junk 2_v2 (Autodesk Fusion 360 design; units mm, degrees)
Autodesk Fusion 360 part; units mm, degrees
note: some values were not read from the file. Chosen so that the rebuilt part matches the saved one: which bodies a step acts on.
sketch "pump stamp sketch" plane through (0, 0, 0) normal (0, 0, 1) x (1, 0, 0)
  circle A0 centre (0, 0) radius 15
  circle A1 centre (-24.5, 0) radius 1.5
  circle A2 centre (-15.5, 15.5) radius 1.5
  circle A3 centre (15.5, 15.5) radius 1.5
  circle A4 centre (-15.5, -15.5) radius 1.5
  circle A5 centre (15.5, -15.5) radius 1.5
  line L0 (-26, 17) -> (26, 17)
  line L1 (26, 17) -> (26, -17)
  line L2 (26, -17) -> (-26, -17)
  line L3 (-26, -17) -> (-26, 17)
  line L4 (-26, 17) -> (26, -17) construction
  line L5 (26, 17) -> (-26, -17) construction
  circle A6 centre (24.5, 0) radius 1.5
  dimension "d569" = 30
  dimension "d570" = 3
  dimension "d576" = 3
  dimension "d579" = 31
  dimension "d580" = -31
  dimension "d581" = 15.5
  dimension "d582" = 15.5
  dimension "d583" = 52
  dimension "d584" = 34
  dimension "d587" = 49
  dimension "d588" = 0
  constraint horizontal A0.centre A1.centre
  constraint coincident A0.centre origin
  constraint horizontal L0
  constraint perpendicular L0 L1
  constraint parallel L0 L2
  constraint parallel L1 L3
  constraint coincident L4 A0.centre
  constraint coincident L5 A0.centre
  constraint tangent L1 A6
  measures "d569" diameter of A0
  measures "d570" diameter of A1
  measures "d576" diameter of A2
  measures "d581" horizontal distance of A0.centre A2.centre
  measures "d582" vertical distance of A0.centre A2.centre
  measures "d583" distance of L0.start L0.end
  measures "d584" distance of L0.start L2.end
extrude "Extrude Pump Stamp" add sketch "pump stamp sketch" along normal blind 4.175 contours A0 | A1 | A4 | A5 | A6 | A3 | A2 makes body 1 at (-14.0075, -15.3506, 2.7833) makes body 2 at (3.6653, 3.4009, 0) makes body 3 at (16.9925, -15.3506, 2.7833) makes body 4 at (-23.0075, -0.1494, 1.3917) makes body 5 at (16.9925, 15.6494, 2.7833) makes body 6 at (25.9925, -0.1494, 2.7833) makes body 7 at (-14.0075, 15.6494, 2.7833)
sketch " minus 1 mm base" plane through (0, 0, 0) normal (0, 0, 1) x (1, 0, 0)
  line L0 (-41.472, 21.911) -> (35.1129, 21.911)
  line L1 (35.1129, 21.911) -> (35.1129, -26.7494)
  line L2 (35.1129, -26.7494) -> (-41.472, -26.7494)
  line L3 (-41.472, -26.7494) -> (-41.472, 21.911)
  dimension "d591" = 76.5849
  constraint horizontal L0
  constraint vertical L1
  constraint horizontal L2
  constraint vertical L3
  measures "d591" distance of L0.start L0.end
extrude "Extrude The minus 1mm base" add sketch " minus 1 mm base" against normal blind 1 bodies 1 7 2 5 4 6 3
copy_body "CopyPasteBodies13" bodies 1 makes body 8
move_body "Move38" bodies 8 to x (1, 0, 0) y (0, 1, 0) z (0, 0, 1) at (100, 0, 0)
sketch "Sketch18" plane through (0, 0, 0) normal (0, 0, 1) x (1, 0, 0)
  line L0 (42.8223, 34.8293) -> (158.9585, 34.8293)
  line L1 (158.9585, 34.8293) -> (158.9585, -31.3539)
  line L2 (158.9585, -31.3539) -> (42.8223, -31.3539)
  line L3 (42.8223, -31.3539) -> (42.8223, 34.8293)
  dimension "d596" = 116.1362
  constraint horizontal L0
  constraint vertical L1
  constraint horizontal L2
  constraint vertical L3
  measures "d596" distance of L0.start L0.end
extrude "Extrude23" cut sketch "Sketch18" against normal blind 1 bodies 8 makes body 9 at (114.3509, -16.4642, 2.7833) makes body 10 at (125.9925, -0.1494, 2.7833) makes body 11 at (76.9925, -0.1494, 1.3917) makes body 12 at (114.6244, 14.2821, 2.7833) makes body 13 at (103.8315, 5.6199, 4.175) makes body 14 at (85.9925, 15.6494, 2.7833)
equation "fingerWidth = 10 mm"
equation "length = 240 mm"
equation "thickness = 3.175 mm"
equation "height = 60 mm"
equation "toolDiameter = 1.401 mm"
equation "boneCornerToCenter = toolDiameter / 2 / sqrt(2) - 0 * kerf" comment "Best: 2.001 -2*kerf, 0.1;;;Best: 2.001 no kerf and 0.1   OLD+6 kerf at 2.001 Diam and .1 mm"
equation "tempLengthPiecesBottom = ceil(( ( floor(( length - 2 * thickness ) / fingerWidth) - 2 ) - ( ( floor(( length - 2 * thickness ) / fingerWidth) - 2 ) % 2 - 1 ) ))"
equation "lengthCutsBottom = ceil(tempLengthPiecesBottom / 2)"
equation "lengthShoulder = ( length - fingerWidth * tempLengthPiecesBottom ) / 2 - kerf"
equation "depth = 185 mm"
equation "tempDepthPiecesBottom = ceil(( ( floor(( depth - 2 * thickness ) / fingerWidth) - 2 ) - ( ( floor(( depth - 2 * thickness ) / fingerWidth) - 2 ) % 2 - 1 ) ))"
equation "depthCutsSideBottom = ceil(tempDepthPiecesBottom / 2)"
equation "depthShoulder = ( depth - fingerWidth * tempDepthPiecesBottom ) / 2 - kerf"
equation "tempHeightPiecesSide = ceil(( ( floor(( height - 2 * thickness ) / fingerWidth) - 2 ) - ( ( floor(( height - 2 * thickness ) / fingerWidth) - 2 ) % 2 - 1 ) ))"
equation "heightCutsSide = ceil(tempHeightPiecesSide / 2)"
equation "heightSholder = ( height - fingerWidth * tempHeightPiecesSide ) / 2 - kerf"
equation "kerf = -0.095 mm"
equation "holeWidth = fingerWidth + 2 * kerf"
equation "lengthShoulderHole = lengthShoulder + 2 * kerf"
equation "depthShouderHole = depthShoulder + 2 * kerf"
equation "heightShoulderHole = heightSholder + 2 * kerf"
equation "assembleScrewDiam = 2.1 mm"
equation "assembleScrewDistance = 6 mm"
equation "assembleAvoidCollisionDistance = 1 mm"
equation "coolingHoleDistance = 8 mm"
equation "boneCornerToCenterPack = -3 * kerf"
equation "boneCornerToCenterSide = boneCornerToCenter - boneCornerToCenterPack"
equation "d589 = thickness + 1 mm"
named bodies: "Pump Stamp", "Pump Stamp (1)", "Pump Stamp (1) (1)", "Pump Stamp (1) (2)", "Pump Stamp (1) (3)", "Pump Stamp (1) (4)", "Pump Stamp (1) (5)", "Pump Stamp (1) (6)"
